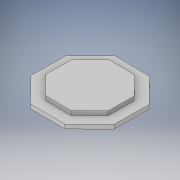
# Autodesk Inventor part: oktagonUnten
Saved by Autodesk Inventor 2019 (Build 230136000, 136)
## iProperties
Created: 2018-08-07
Part Number: oktagonUnten
Material: Generic
Document SubType Name: Modeling
Designer: chris
Density: 1 g/cm^3
Appearance: Default
Author: chris
Autodesk Inventor part; units mm, degrees
ref_plane "YZ Plane" through (0, 0, 0) normal (1, 0, 0) x (0, 1, 0)
ref_plane "XZ Plane" through (0, 0, 0) normal (0, 1, 0) x (-1, 0, 0)
ref_plane "XY Plane" through (0, 0, 0) normal (0, 0, 1) x (1, 0, 0)
sketch "Sketch1" plane through (0, 0, 0) normal (0, 1, 0) x (-1, 0, 0)
  line L0 (20.0643, 8.1272) -> (19.9344, -8.4408)
  line L1 (19.9344, -8.4408) -> (8.1272, -20.0643)
  line L2 (8.1272, -20.0643) -> (-8.4408, -19.9344)
  line L3 (-8.4408, -19.9344) -> (-20.0643, -8.1272)
  line L4 (-20.0643, -8.1272) -> (-19.9344, 8.4408)
  line L5 (-19.9344, 8.4408) -> (-8.1272, 20.0643)
  line L6 (-8.1272, 20.0643) -> (8.4408, 19.9344)
  line L7 (8.4408, 19.9344) -> (20.0643, 8.1272)
  point P0 (0, 0)
  point P1 (0, 0)
  dimension "d0" = 20
  dimension "d1" = 16.568
  constraints: 16 end point, 1 coincident, 17 other
  measures "d0" distance from line of L0 point (0, 0)
  measures "d1" vertical distance of L3.end L4.end
extrude "Extrusion1" add sketch "Sketch1" along normal blind 2
sketch "Sketch2" plane through (0, 2, 0) normal (0, 1, 0) x (1, 0, 0)
  line L0 (15.0642, 6.0559) -> (14.9342, -6.3698)
  line L1 (14.9342, -6.3698) -> (6.0559, -15.0642)
  line L2 (6.0559, -15.0642) -> (-6.3698, -14.9342)
  line L3 (-6.3698, -14.9342) -> (-15.0642, -6.0559)
  line L4 (-15.0642, -6.0559) -> (-14.9342, 6.3698)
  line L5 (-14.9342, 6.3698) -> (-6.0559, 15.0642)
  line L6 (-6.0559, 15.0642) -> (6.3698, 14.9342)
  line L7 (6.3698, 14.9342) -> (15.0642, 6.0559)
  point P0 (0, 0)
  point P1 (0, 0)
  dimension "d4" = 15
  dimension "d5" = 12.4257
  constraints: 16 end point, 1 coincident, 17 other
  measures "d4" distance from line of L0 point (0, 0)
  measures "d5" vertical distance of L3.end L4.end
extrude "Extrusion2" add sketch "Sketch2" along normal blind 2
body "Solid1"
